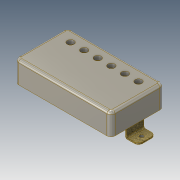
# Autodesk Inventor part: capacitor
Saved by Autodesk Inventor 2016 (Build 200138000, 138)
## iProperties
Created: 2018-12-07
Part Number: capacitor
Material: Titanium
Document SubType Name: Modeling
Designer: lesly
Density: 4.51 g/cm^3
Appearance: Titanium - Polished
Author: lesly
Autodesk Inventor part; units mm, degrees
ref_plane "YZ Plane" through (0, 0, 0) normal (1, 0, 0) x (0, 1, 0)
ref_plane "XZ Plane" through (0, 0, 0) normal (0, 1, 0) x (-1, 0, 0)
ref_plane "XY Plane" through (0, 0, 0) normal (0, 0, 1) x (1, 0, 0)
sketch "Sketch1" plane through (0, 0, 0) normal (0, 1, 0) x (-1, 0, 0)
  line L0 (9.0772, 19.5) -> (-61.9228, 19.5)
  line L1 (-61.9228, 19.5) -> (-61.9228, -19.5)
  line L2 (-61.9228, -19.5) -> (9.0772, -19.5)
  line L3 (9.0772, -19.5) -> (9.0772, 19.5)
  point P0 (0, 0)
  dimension "d0" = 71
  dimension "d1" = 39
  dimension "d147" = 19.5
  constraints: 8 end point, 2 parallel, 1 horizontal, 1 perpendicular
  measures "d0" distance of L2.end L1.end
  measures "d1" distance of L1.end L0.end
  measures "d147" distance from line of L2 point (0, 0)
extrude "Extrusion1" add sketch "Sketch1" along normal mid plane 16
fillet "Fillet1" radius 2 4 edges at (26.4228, 8, 19.5) (-9.0772, 8, 0) (26.4228, 8, -19.5) (61.9228, 8, 0)
fillet "Fillet2" radius 3 2 edges at (61.9228, -1, 19.5) (61.3371, 7.4142, 18.9142)
fillet "Fillet3" radius 3 2 edges at (61.3371, 7.4142, -18.9142) (61.9228, -1, -19.5)
fillet "Fillet4" radius 3 2 edges at (-8.4914, 7.4142, 18.9142) (-9.0772, -1, 19.5)
fillet "Fillet5" radius 3 2 edges at (-8.4914, 7.4142, -18.9142) (-9.0772, -1, -19.5)
sketch "Sketch2" plane through (0, -8, 0) normal (0, -1, 0) x (1, 0, 0)
  arc A0 (58.9228, -19.5) -> (61.9228, -16.5) centre (58.9228, -16.5) ccw
  line L0 (-7.0772, -16.5) -> (-7.0772, 15.5)
  arc A1 (-5.0772, 17.5) -> (-7.0772, 15.5) centre (-5.0772, 15.5) ccw
  arc A2 (60.9228, 15.5) -> (58.9228, 17.5) centre (58.9228, 15.5) ccw
  line L1 (60.9228, 15.5) -> (60.9228, -16.5)
  arc A3 (58.9228, -18.5) -> (60.9228, -16.5) centre (58.9228, -16.5) ccw
  arc A4 (-7.0772, -16.5) -> (-5.0772, -18.5) centre (-5.0772, -16.5) ccw
  line L2 (-1.0772, -18.5) -> (-1.0772, -19.5)
  line L3 (-1.0772, 17.5) -> (-1.0772, 18.5)
  line L4 (54.9236, -18.5) -> (54.9236, -19.5)
  line L5 (58.9228, -18.5) -> (54.9236, -18.5)
  line L6 (-1.0772, -18.5) -> (-5.0772, -18.5)
  line L7 (-5.0772, 17.5) -> (-1.0772, 17.5)
  line L8 (54.9236, 17.5) -> (58.9228, 17.5)
  line L9 (54.9236, -19.5) -> (54.9236, -18.5)
  line L10 (54.9236, 17.5) -> (54.9236, 18.5)
  line L11 (-1.0772, -19.5) -> (54.9236, -19.5)
  line L12 (-1.0772, 17.5) -> (54.9236, 17.5)
  line L13 (-1.0772, -18.5) -> (54.9236, -18.5)
  line L14 (-6.0772, -17.5) -> (58.9228, -17.5) projected
  point P0 (0, 0)
  point P1 (-9.0772, 16.5)
  point P2 (58.9228, 19.5)
  constraints: 28 end point, 10 point on circle, 6 parallel, 5 centre point, 4 perpendicular, 1 collinear, 1 point on line
extrude "Extrusion2" add sketch "Sketch2" along normal blind 1 contours L0 A1 L7 L12 L8 A2 L1 A3 L5 L13 L6 A4
fillet "Fillet6" radius 0.5 8 edges at (-6.4914, -9, 16.9142) (-7.0772, -9, -0.5) (-6.4914, -9, -17.9142) (26.9228, -9, -18.5) (60.3371, -9, -17.9142) (60.9228, -9, -0.5) (60.3371, -9, 16.9142) (26.9228, -9, 17.5)
sketch "Sketch3" plane through (0, 0, 0) normal (0, 0, 1) x (1, 0, 0)
  line L0 (60.4228, -9) -> (58.9228, -9) projected
  line L1 (60.4228, -9) -> (60.4228, -14)
  line L2 (60.4228, -9) -> (59.4228, -9)
  line L3 (59.4228, -9) -> (59.4228, -15)
  line L4 (60.4228, -16) -> (68.9228, -16)
  line L5 (68.9228, -16) -> (68.9228, -15)
  line L6 (68.9228, -15) -> (61.4228, -15)
  arc A0 (59.4228, -15) -> (60.4228, -16) centre (60.4228, -15) ccw
  arc A1 (60.4228, -14) -> (61.4228, -15) centre (61.4228, -14) ccw
  line L7 (58.9228, 8) -> (-6.0772, 8) projected
  line L8 (-7.0772, -9) -> (-5.0772, -9)
  line L9 (-7.0772, -9) -> (-7.0772, -14)
  line L10 (-7.0772, -9) -> (-6.0772, -9)
  line L11 (-6.0772, -9) -> (-6.0772, -15)
  line L12 (-7.0772, -16) -> (-15.0772, -16)
  line L13 (-15.0772, -16) -> (-15.0772, -15)
  line L14 (-15.0772, -15) -> (-8.0772, -15)
  arc A2 (-7.0772, -16) -> (-6.0772, -15) centre (-7.0772, -15) ccw
  arc A3 (-8.0772, -15) -> (-7.0772, -14) centre (-8.0772, -14) ccw
  line L15 (58.9228, -9) -> (-5.0772, -9) projected
  line L16 (26.9228, -9) -> (26.9228, -14.7071) construction
  point P0 (0, 0)
  point P1 (59.4228, -16)
  point P2 (-6.0772, -16)
  dimension "d133" = 84
  dimension "d134" = 42
  constraints: 28 end point, 8 point on circle, 5 point on line, 4 centre point, 4 tangent, 3 vertical, 2 midpoint, 2 perpendicular, 1 horizontal
  measures "d133" distance of L4.end L12.end
  measures "d134" distance from line of L16 L12.end
extrude "Extrusion3" add sketch "Sketch3" along normal mid plane 12.5
fillet "Fillet7" radius 3 2 edges at (-15.0772, -15.5, 6.25) (-15.0772, -15.5, -6.25)
fillet "Fillet8" radius 3 2 edges at (68.9228, -15.5, 6.25) (68.9228, -15.5, -6.25)
sketch "Sketch5" plane through (0, 8, 0) normal (0, 1, 0) x (1, 0, 0)
  line L0 (-9.0772, -16.5) -> (-9.0772, 16.5) projected
  line L1 (61.9228, -16.5) -> (61.9228, 16.5) projected
  circle A0 centre (51.9228, 10.7251) radius 2.5
  circle A1 centre (41.9228, 10.7251) radius 2.5
  circle A2 centre (31.9228, 10.7251) radius 2.5
  circle A3 centre (21.9228, 10.7251) radius 2.5
  circle A4 centre (11.9228, 10.7251) radius 2.5
  circle A5 centre (1.9228, 10.7251) radius 2.5
  point P0 (0, 0)
  constraints: 6 centre point
sketch "Sketch6" plane through (-8.0772, -15, 6.25) normal (0, 1, 0) x (1, 0, 0)
  line L0 (-7, 9.5) -> (-7, 3) construction
  circle A0 centre (-4, 6.25) radius 1.5
  line L1 (2, -13.25) -> (67, -13.25) construction
  line L2 (67, 25.75) -> (2, 25.75) construction
  circle A1 centre (73, 6.25) radius 1.5
  line L3 (67, -13.25) -> (2, -13.25) construction
  line L4 (34.5, -13.25) -> (34.5, -15.2484) construction
  line L5 (67, 25.75) -> (2, 25.75) construction
  line L6 (2, -13.25) -> (67, -13.25) construction
  line L7 (70, -10.25) -> (70, 22.75) projected
  line L8 (-1, 22.75) -> (-1, -10.25) projected
  point P0 (8.0772, 6.25)
  dimension "d109" = 3
  dimension "d110" = 3
  dimension "d135" = 77
  dimension "d136" = 38.5
  dimension "d140" = 39
  dimension "d141" = 71
  dimension "d142" = 19.5
  dimension "d143" = 19.5
  dimension "d144" = 19.5
  dimension "d145" = 19.5
  dimension "d146" = 38.5
  dimension "d148" = 19.5
  constraints: 12 end point, 2 centre point, 1 midpoint, 1 vertical, 1 other
  measures "d109" diameter of A1
  measures "d110" diameter of A0
  measures "d135" distance of A1.centre A0.centre
  measures "d136" distance from line of A0.centre L4
  measures "d140" distance between parallel lines of L2 L1
  measures "d141" distance between parallel lines of L7 L8
  measures "d142" distance from line of L1 A0.centre
  measures "d143" distance from line of L2 A0.centre
  measures "d144" distance from line of L3 A1.centre
  measures "d145" distance from line of L2 A1.centre
  measures "d146" horizontal distance of A1.centre L4.end
  measures "d148" distance from line of L1 point (8.077, 6.25)
extrude "Extrusion4" cut sketch "Sketch6" against normal blind 12.5
hole "Hole1" at (51.9228, 8, -10.7251) at (41.9228, 8, -10.7251) at (31.9228, 8, -10.7251) at (21.9228, 8, -10.7251) at (11.9228, 8, -10.7251) at (1.9228, 8, -10.7251) direction (0, -1, 0) diameter 3 depth 21 counterbore diameter 5 counterbore depth 3
sketch "Sketch7" plane through (0, -9, 0) normal (0, -1, 0) x (1, 0, 0)
  circle A0 centre (31.9228, -10.7251) radius 1.5 projected
  circle A1 centre (11.9228, -10.7251) radius 1.5 projected
  circle A2 centre (1.9228, -10.7251) radius 1.5 projected
  circle A3 centre (51.9228, -10.7251) radius 1.5 projected
  circle A4 centre (51.9228, 7.2749) radius 1.5
  circle A5 centre (1.9228, 7.2749) radius 1.5
  circle A6 centre (41.9228, -10.7251) radius 1.5 projected
  circle A7 centre (21.9228, -10.7251) radius 1.5 projected
  circle A8 centre (41.9228, 7.2749) radius 1.5
  circle A9 centre (31.9228, 7.2749) radius 1.5
  circle A10 centre (21.9228, 7.2749) radius 1.5
  circle A11 centre (11.9228, 7.2749) radius 1.5
  point P0 (0, 0)
  constraints: 6 centre point
extrude "Extrusion5" cut sketch "Sketch7" against normal blind 1 contours A4 | A5 | A8 | A9 | A10 | A11
sketch "Sketch8" plane through (0, -9, 0) normal (0, -1, 0) x (1, 0, 0)
  line L0 (58.9228, -18) -> (-5.0772, -18) projected
  line L1 (-0.643, -14.134) -> (-2.1755, -14.1094)
  line L2 (-2.2313, -17.5769) -> (-0.6988, -17.6015)
  arc A0 (-0.6988, -17.6015) -> (-0.643, -14.134) centre (-0.6709, -15.8678) ccw
  arc A1 (-2.1755, -14.1094) -> (-2.2313, -17.5769) centre (-2.2034, -15.8431) ccw
  line L3 (57.028, 14.4029) -> (55.4956, 14.4275)
  line L4 (55.4398, 10.96) -> (56.9723, 10.9354)
  arc A2 (56.9723, 10.9354) -> (57.028, 14.4029) centre (57.0002, 12.6692) ccw
  arc A3 (55.4956, 14.4275) -> (55.4398, 10.96) centre (55.4677, 12.6938) ccw
  point P0 (0, 0)
  point P1 (-2.321, -18.5267)
  constraints: 8 end point, 8 point on circle, 8 tangent, 4 centre point, 2 parallel
extrude "Extrusion6" cut sketch "Sketch8" against normal blind 15
sketch "Sketch9" plane through (-7.0772, -16, -6.25) normal (0, -1, 0) x (1, 0, 0)
  circle A0 centre (-5, 6.25) radius 1.5
  circle A1 centre (-5, 6.25) radius 2
  line L0 (1, -13.25) -> (66, -13.25) construction
  circle A2 centre (72, 6.25) radius 1.5
  circle A3 centre (72, 6.25) radius 2
  line L1 (66, 25.75) -> (1, 25.75) construction
  line L2 (33.5, 25.75) -> (33.5, 16.5004) construction
  circle A4 centre (-5, 7.25) radius 1.5 construction
  circle A5 centre (72, 7.25) radius 1.5 construction
  point P0 (7.0772, 6.25)
  dimension "d105" = 4
  dimension "d111" = 3
  dimension "d112" = 3
  dimension "d137" = 77
  dimension "d138" = 38.5
  dimension "d139" = 38.5
  constraints: 6 centre point, 2 coincident, 2 end point, 1 midpoint, 1 vertical
  measures "d105" diameter of A1
  measures "d111" diameter of A2
  measures "d112" diameter of A0
  measures "d137" distance of A2.centre A0.centre
  measures "d138" horizontal distance of A0.centre L2.end
  measures "d139" horizontal distance of A2.centre L2.end
extrude "Extrusion7" add sketch "Sketch9" along normal blind 1
thread "Thread1" size "M3x0.35" class "6H" standard "ANSI Metric M Profile" full length
thread "Thread2" size "M3x0.35" class "6H" standard "ANSI Metric M Profile" full length
thread "Thread3" size "M3x0.35" class "6H" standard "ANSI Metric M Profile" full length
thread "Thread4" size "M3x0.35" class "6H" standard "ANSI Metric M Profile" full length
thread "Thread5" size "M3x0.35" class "6H" standard "ANSI Metric M Profile" full length
thread "Thread6" size "M3x0.35" class "6H" standard "ANSI Metric M Profile" full length
thread "Thread7" size "M3x0.35" class "6H" standard "ANSI Metric M Profile" full length
thread "Thread8" size "M3x0.35" class "6H" standard "ANSI Metric M Profile" full length
thread "Thread9" size "M3x0.35" class "6H" standard "ANSI Metric M Profile" full length
thread "Thread10" size "M3x0.35" class "6H" standard "ANSI Metric M Profile" full length
body "Solid1"
